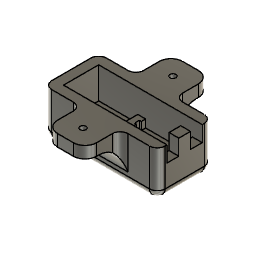
ATtiny85 LED Controller (Autodesk Fusion 360 design; units mm, degrees)
Autodesk Fusion 360 part; units mm, degrees
sketch "Sketch6" plane through (0, 0, 0) normal (0, 0, 1) x (1, 0, 0)
  line L0 (0, 0) -> (24, 0)
  line L1 (24, 0) -> (24, 9)
  line L2 (24, 9) -> (0, 9)
  line L3 (0, 9) -> (0, 0)
  line L4 (24, 9) -> (26.5, 9) construction
  line L5 (26.5, 9) -> (26.5, 11.5) construction
  line L6 (0, 0) -> (-2.5, 0) construction
  line L7 (-2.5, 0) -> (-2.5, -2.5) construction
  line L8 (26.5, 11.5) -> (-2.5, 11.5)
  line L9 (-2.5, 11.5) -> (-2.5, -2.5)
  line L10 (-2.5, -2.5) -> (26.5, -2.5)
  line L11 (26.5, -2.5) -> (26.5, 11.5)
  dimension "d28" = 24
  dimension "d29" = 9
  dimension "d32" = 2.5
  dimension "d33" = 2.5
  dimension "d34" = 2.5
  dimension "d35" = 2.5
  constraint horizontal L0
  constraint vertical L1
  constraint horizontal L2
  constraint vertical L3
  constraint coincident L0.start L3.end
  constraint perpendicular L1 L4
  constraint perpendicular L4 L5
  constraint perpendicular L3 L6
  constraint perpendicular L6 L7
  constraint horizontal L8
  constraint vertical L9
  constraint horizontal L10
  constraint vertical L11
  measures "d28" distance of L0.start L0.end
  measures "d29" distance of L0.start L2.end
  measures "d32" distance of L1.end L4.end
  measures "d33" distance of L4.end L5.end
  measures "d34" distance of L0.start L6.end
  measures "d35" distance of L6.end L7.end
extrude "Extrude8" add sketch "Sketch6" along normal blind 3.5 contours L0 L1 L2 L3
sketch "Sketch7" plane through (0, 0, 3.5) normal (0, 0, 1) x (-1, 0, 0)
  line L0 (0, -9) -> (0, 0)
  line L1 (0, 0) -> (-24, 0)
  line L2 (-24, 0) -> (-24, -9)
  line L3 (-24, -9) -> (0, -9)
  line L4 (-12, -9) -> (-10, -9)
  line L5 (-10, -9) -> (-10, 0)
  line L6 (-10, 0) -> (-12, 0)
  line L7 (-12, 0) -> (-12, -9)
  constraint horizontal L4
  constraint vertical L5
  constraint horizontal L6
  constraint vertical L7
  constraint midpoint L3 L4.start
extrude "Extrude9" add sketch "Sketch7" along normal blind 2 contours L1 L3 L4 L5 L6 L7
sketch "Sketch8" plane through (0, 0, 0) normal (0, 0, -1) x (1, 0, 0)
  line L0 (0, 0) -> (0, -9)
  line L1 (0, -9) -> (24, -9)
  line L2 (24, -9) -> (24, 0)
  line L3 (24, 0) -> (0, 0)
  line L4 (12, 0) -> (12, -9) construction
  line L5 (15.4, -7.9) -> (8.6, -7.9)
  line L6 (8.6, -7.9) -> (8.6, -1.1)
  line L7 (8.6, -1.1) -> (15.4, -1.1)
  line L8 (15.4, -1.1) -> (15.4, -7.9)
  line L9 (15.4, -7.9) -> (8.6, -1.1) construction
  line L10 (8.6, -7.9) -> (15.4, -1.1) construction
  point P0 (12, -4.5)
  dimension "d39" = 6.8
  dimension "d40" = 6.8
  constraint midpoint L3 L4.start
  constraint midpoint L1 L4.end
  constraint horizontal L5
  constraint perpendicular L5 L6
  constraint parallel L5 L7
  constraint parallel L6 L8
  constraint coincident L9 P0
  constraint coincident L10 P0
  constraint midpoint L4 P0
  measures "d39" distance of L6.end L7.end
  measures "d40" distance of L5.end L6.end
extrude "Extrude10" cut sketch "Sketch8" against normal blind 3 contours L5 L6 L7 L8
extrude "Extrude13" add sketch "Sketch6" along normal blind 11.5
sketch "Sketch10" plane through (0, 0, 11.5) normal (0, 0, 1) x (-1, 0, 0)
  line L0 (0, 0) -> (0, -9)
  line L1 (0, -9) -> (-24, -9)
  line L2 (-24, -9) -> (-24, 0)
  line L3 (-24, 0) -> (0, 0)
  line L4 (-26.5, 2.5) -> (-26.5, -11.5)
  line L5 (-26.5, -11.5) -> (2.5, -11.5)
  line L6 (2.5, -11.5) -> (2.5, 2.5)
  line L7 (2.5, 2.5) -> (-26.5, 2.5)
  line L8 (-24, 0) -> (-26.5, 0)
  line L9 (-26.5, 0) -> (-26.5, -3)
  line L10 (-26.5, -3) -> (-24, -3)
  line L11 (-24, -3) -> (-24, 0)
  line L12 (-24, -9) -> (-26.5, -9)
  line L13 (-26.5, -9) -> (-26.5, -6)
  line L14 (-26.5, -6) -> (-24, -6)
  line L15 (-24, -6) -> (-24, -9)
  dimension "d50" = 3
  dimension "d51" = 3
  constraint horizontal L8
  constraint vertical L9
  constraint horizontal L10
  constraint vertical L11
  constraint coincident L2.end L3.start
  constraint horizontal L12
  constraint vertical L13
  constraint horizontal L14
  constraint vertical L15
  constraint coincident L1.end L2.start
  measures "d50" distance of L2.end L10.end
  measures "d51" distance of L1.end L14.end
extrude "Extrude14" cut sketch "Sketch10" against normal blind 4 contours L2 L4 L8 L9 L10 L11 | L2 L4 L12 L13 L14 L15
sketch "Sketch11" plane through (0, 11.5, 0) normal (0, 1, 0) x (-1, 0, 0)
  line L0 (-26.5, 0) -> (2.5, 0)
  line L1 (2.5, 0) -> (2.5, 11.5)
  line L2 (2.5, 11.5) -> (-26.5, 11.5)
  line L3 (-26.5, 11.5) -> (-26.5, 0)
  line L4 (-12, 11.5) -> (-7, 11.5) construction
  line L5 (-7, 11.5) -> (-17, 11.5)
  line L6 (-17, 11.5) -> (-17, 8.5)
  line L7 (-17, 8.5) -> (-7, 8.5)
  line L8 (-7, 8.5) -> (-7, 11.5)
  dimension "d54" = 5
  dimension "d55" = 10
  dimension "d56" = 3
  constraint midpoint L2 L4.start
  constraint parallel L2 L4
  constraint horizontal L5
  constraint vertical L6
  constraint horizontal L7
  constraint vertical L8
  measures "d54" distance of L4.start L4.end
  measures "d55" distance of L4.end L5.end
  measures "d56" distance of L4.end L7.end
extrude "Extrude15" add sketch "Sketch11" along normal blind 9 contours L2 L5 L6 L7 L8
sketch "Sketch12" plane through (0, -2.5, 0) normal (0, -1, 0) x (1, 0, 0)
  line L0 (-2.5, 0) -> (26.5, 0)
  line L1 (26.5, 0) -> (26.5, 11.5)
  line L2 (26.5, 11.5) -> (-2.5, 11.5)
  line L3 (-2.5, 11.5) -> (-2.5, 0)
  line L4 (12, 11.5) -> (17, 11.5) construction
  line L5 (17, 11.5) -> (7, 11.5)
  line L6 (7, 11.5) -> (7, 8.5)
  line L7 (7, 8.5) -> (17, 8.5)
  line L8 (17, 8.5) -> (17, 11.5)
  dimension "d59" = 5
  dimension "d60" = 10
  dimension "d61" = 3
  constraint midpoint L2 L4.start
  constraint parallel L2 L4
  constraint horizontal L5
  constraint vertical L6
  constraint horizontal L7
  constraint vertical L8
  measures "d59" distance of L4.start L4.end
  measures "d60" distance of L4.end L5.end
  measures "d61" distance of L4.end L7.end
extrude "Extrude16" add sketch "Sketch12" along normal blind 9 contours L2 L5 L6 L7 L8
fillet "Fillet1" radius 5.5 2 edges at (12, -2.5, 8.5) (12, 11.5, 8.5)
fillet "Fillet2" radius 3 4 edges at (17, 20.5, 10) (7, 20.5, 10) (17, -11.5, 10) (7, -11.5, 10)
fillet "Fillet3" radius 2 4 edges at (-2.5, 11.5, 5.75) (-2.5, -2.5, 5.75) (26.5, 11.5, 5.75) (26.5, -2.5, 5.75)
fillet "Fillet4" radius 2 4 edges at (7, -2.5, 7.25) (17, -2.5, 7.25) (17, 11.5, 7.25) (7, 11.5, 7.25)
sketch "Sketch13" plane through (0, 0, 11.5) normal (0, 0, 1) x (-1, 0, 0)
  arc A0 (-24.5, 2.5) -> (-26.5, 0.5) centre (-24.5, 0.5) ccw
  line L0 (-26.5, 0.5) -> (-26.5, 0)
  line L1 (-26.5, 0) -> (0, 0)
  line L2 (0, 0) -> (0, -9)
  line L3 (0, -9) -> (-26.5, -9)
  line L4 (-26.5, -9) -> (-26.5, -9.5)
  arc A1 (-26.5, -9.5) -> (-24.5, -11.5) centre (-24.5, -9.5) ccw
  line L5 (-24.5, -11.5) -> (-19, -11.5)
  arc A2 (-17, -13.5) -> (-19, -11.5) centre (-19, -13.5) ccw
  line L6 (-17, -13.5) -> (-17, -17.5)
  arc A3 (-17, -17.5) -> (-14, -20.5) centre (-14, -17.5) ccw
  line L7 (-14, -20.5) -> (-10, -20.5)
  arc A4 (-10, -20.5) -> (-7, -17.5) centre (-10, -17.5) ccw
  line L8 (-7, -17.5) -> (-7, -13.5)
  arc A5 (-5, -11.5) -> (-7, -13.5) centre (-5, -13.5) ccw
  line L9 (-5, -11.5) -> (0.5, -11.5)
  arc A6 (0.5, -11.5) -> (2.5, -9.5) centre (0.5, -9.5) ccw
  line L10 (2.5, -9.5) -> (2.5, 0.5)
  arc A7 (2.5, 0.5) -> (0.5, 2.5) centre (0.5, 0.5) ccw
  line L11 (0.5, 2.5) -> (-5, 2.5)
  arc A8 (-7, 4.5) -> (-5, 2.5) centre (-5, 4.5) ccw
  line L12 (-7, 4.5) -> (-7, 8.5)
  arc A9 (-7, 8.5) -> (-10, 11.5) centre (-10, 8.5) ccw
  line L13 (-10, 11.5) -> (-14, 11.5)
  arc A10 (-14, 11.5) -> (-17, 8.5) centre (-14, 8.5) ccw
  line L14 (-17, 8.5) -> (-17, 4.5)
  arc A11 (-19, 2.5) -> (-17, 4.5) centre (-19, 4.5) ccw
  line L15 (-19, 2.5) -> (-24.5, 2.5)
  line L16 (-12, -20.5) -> (-12, -16) construction
  line L17 (-12, 11.5) -> (-12, 7) construction
  circle A12 centre (-12, -16) radius 0.75
  circle A13 centre (-12, 7) radius 0.75
  dimension "d72" = 4.5
  dimension "d73" = 1.5
  dimension "d74" = 1.5
  constraint midpoint L7 L16.start
  constraint perpendicular L7 L16
  constraint midpoint L13 L17.start
  constraint perpendicular L13 L17
  constraint coincident L16.end A12.centre
  constraint coincident L17.end A13.centre
  measures "d72" distance of L16.start L16.end
  measures "d73" diameter of A12
  measures "d74" diameter of A13
extrude "Extrude17" cut sketch "Sketch13" against normal blind 5 contours A12 | A13
sketch "Sketch14" plane through (0, 0, 3) normal (0, 0, -1) x (1, 0, 0)
  line L0 (15.4, -1.1) -> (8.6, -1.1)
  line L1 (8.6, -1.1) -> (8.6, -7.9)
  line L2 (8.6, -7.9) -> (15.4, -7.9)
  line L3 (15.4, -7.9) -> (15.4, -1.1)
  line L4 (12, -1.1) -> (12.5, -1.1)
  line L5 (12.5, -1.1) -> (11.5, -1.1)
  line L6 (11.5, -1.1) -> (11.5, -2.3)
  line L7 (11.5, -2.3) -> (12.5, -2.3)
  line L8 (12.5, -2.3) -> (12.5, -1.1)
  line L9 (12, -7.9) -> (11.5, -7.9)
  line L10 (11.5, -7.9) -> (12.5, -7.9)
  line L11 (12.5, -7.9) -> (12.5, -6.7)
  line L12 (12.5, -6.7) -> (11.5, -6.7)
  line L13 (11.5, -6.7) -> (11.5, -7.9)
  dimension "d77" = 0.5
  dimension "d78" = 1
  dimension "d79" = 1.2
  dimension "d80" = 0.5
  dimension "d81" = 1
  dimension "d82" = 1.2
  constraint midpoint L0 L4.start
  constraint parallel L0 L4
  constraint horizontal L5
  constraint vertical L6
  constraint horizontal L7
  constraint vertical L8
  constraint midpoint L2 L9.start
  constraint parallel L2 L9
  constraint horizontal L10
  constraint vertical L11
  constraint horizontal L12
  constraint vertical L13
  measures "d77" distance of L4.start L4.end
  measures "d78" distance of L4.end L5.end
  measures "d79" distance of L4.end L7.end
  measures "d80" distance of L9.start L9.end
  measures "d81" distance of L9.end L10.end
  measures "d82" distance of L9.end L12.end
extrude "Extrude18" cut sketch "Sketch14" against normal up to surface (2.5 mm away) contours L0 L4 L5 L6 L7 L8 | L2 L9 L10 L11 L12 L13
fillet "Fillet5" radius 2 8 edges at (12, -2.5, 0) (25.9142, -1.9142, 0) (26.5, 4.5, 0) (25.9142, 10.9142, 0) (12, 11.5, 0) (-1.9142, 10.9142, 0) (-2.5, 4.5, 0) (-1.9142, -1.9142, 0)
